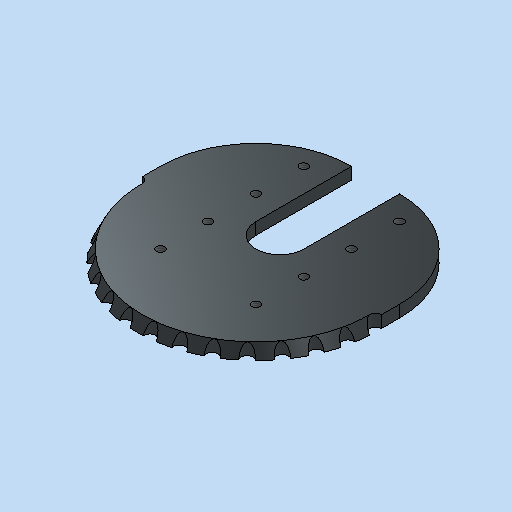
# Autodesk Inventor part: Blade
Saved by Autodesk Inventor 2026.1 (Build 301233000, 233)
## iProperties
Created: 2026-04-14
Part Number: Blade
Material: Iron, Gray
Document SubType Name: Modeling
Designer: ADMIN
Density: 7.15 g/cm^3
Appearance: Iron Gray
Author: ADMIN
Autodesk Inventor part; units mm, degrees
ref_plane "YZ Plane" through (0, 0, 0) normal (1, 0, 0) x (0, 1, 0)
ref_plane "XZ Plane" through (0, 0, 0) normal (0, 1, 0) x (-1, 0, 0)
ref_plane "XY Plane" through (0, 0, 0) normal (0, 0, 1) x (1, 0, 0)
sketch "Sketch1" plane through (0, 0, 0) normal (0, 1, 0) x (-1, 0, 0)
  line L0 (-10, -50) -> (10, -50)
  line L1 (50, -10) -> (50, 0)
  line L2 (0, 50) -> (0, 50)
  line L3 (-50, 0) -> (-50, -10)
  line L4 (-50, -50) -> (50, 50) construction
  line L5 (50, -50) -> (-50, 50) construction
  line L6 (-10, -50) -> (10, -50)
  line L7 (10, -50) -> (10, 0)
  line L8 (10, 0) -> (-10, 0)
  line L9 (-10, 0) -> (-10, -50)
  arc A0 (50, 0) -> (0, 50) centre (0, 0) ccw
  arc A1 (0, 50) -> (-50, 0) centre (0, 0) ccw
  arc A2 (10, -50) -> (50, -10) centre (10, -10) ccw
  arc A3 (-50, -10) -> (-10, -50) centre (-10, -10) ccw
  arc A4 (-50, -2.5) -> (-49.9375, 2.4992) centre (-50, 0) ccw
  line L10 (84.4975, 0) -> (-84.4975, 0) projected
  arc A5 (-49.4272, 7.9502) -> (-48.3266, 12.8272) centre (-48.9074, 10.3956) ccw
  arc A6 (-46.6941, 18.053) -> (-44.6037, 22.5946) centre (-45.6773, 20.3368) ccw
  arc A7 (-41.9203, 27.3667) -> (-38.9313, 31.3744) centre (-40.4508, 29.3893) ccw
  arc A8 (-35.3144, 35.4844) -> (-31.5574, 38.7831) centre (-33.4565, 37.1572) ccw
  arc A9 (-27.1651, 42.0513) -> (-22.8044, 44.4968) centre (-25, 43.3013) ccw
  arc A10 (-17.8285, 46.7803) -> (-13.0546, 48.2657) centre (-15.4508, 47.5528) ccw
  arc A11 (-7.7127, 49.4648) -> (-2.7344, 49.9252) centre (-5.2264, 49.7261) ccw
  arc A12 (2.7401, 49.9874) -> (7.7054, 49.4027) centre (5.2264, 49.7261) ccw
  arc A13 (13.0732, 48.3254) -> (17.8084, 46.7211) centre (15.4508, 47.5528) ccw
  arc A14 (22.8349, 44.5513) -> (27.1331, 41.9975) centre (25, 43.3013) ccw
  arc A15 (31.5987, 38.8301) -> (35.272, 35.4385) centre (33.4565, 37.1572) ccw
  arc A16 (38.9814, 31.4118) -> (41.8693, 27.3306) centre (40.4508, 29.3893) ccw
  arc A17 (44.6604, 22.6207) -> (46.6367, 18.0283) centre (45.6773, 20.3368) ccw
  arc A18 (48.3876, 12.841) -> (49.3659, 7.938) centre (48.9074, 10.3956) ccw
  arc A19 (50, 2.5) -> (49.9375, -2.4992) centre (50, 0) ccw
  circle A20 centre (20, -40) radius 1.75
  circle A21 centre (20, -20) radius 1.75
  circle A22 centre (20, 0) radius 1.75
  circle A23 centre (20, 20) radius 1.75
  line L11 (0, 50) -> (0, -50) construction
  circle A24 centre (-20, -40) radius 1.75
  circle A25 centre (-20, -20) radius 1.75
  circle A26 centre (-20, 0) radius 1.75
  circle A27 centre (-20, 20) radius 1.75
  line L12 (49.9375, -2.4992) -> (50, -2.4992)
  point P0 (0, 0)
  point P1 (47.5, 0)
  point P2 (49.9375, 2.4992)
  point P3 (49.3659, 7.938)
  point P4 (48.3266, 12.8272)
  point P5 (46.6367, 18.0283)
  point P6 (44.6037, 22.5946)
  point P7 (41.8693, 27.3306)
  point P8 (38.9313, 31.3744)
  point P9 (35.272, 35.4385)
  point P10 (31.5574, 38.7831)
  point P11 (27.1331, 41.9975)
  point P12 (22.8044, 44.4968)
  point P13 (17.8084, 46.7211)
  point P14 (13.0546, 48.2657)
  point P15 (2.7344, 49.9252)
  point P16 (0, 50)
  point P17 (-2.7344, 49.9252)
  point P18 (-7.7054, 49.4027)
  point P19 (-13.0546, 48.2657)
  point P20 (-17.8084, 46.7211)
  point P21 (-22.8044, 44.4968)
  point P22 (-27.1331, 41.9975)
  point P23 (-35.272, 35.4385)
  point P24 (-41.8693, 27.3306)
  point P25 (-44.6037, 22.5946)
  point P26 (-46.6367, 18.0283)
  point P27 (-48.3266, 12.8272)
  point P28 (-49.3659, 7.938)
  dimension "d0" = 100
  dimension "d1" = 100
  dimension "d2" = 20
  dimension "d3" = 50
  dimension "d4" = 50
  dimension "d5" = 40
  dimension "d6" = 5
  dimension "d9" = 180
  dimension "d11" = 3.5
  dimension "d12" = 3.5
  dimension "d13" = 3.5
  dimension "d14" = 3.5
  dimension "d15" = 20
  dimension "d16" = 20
  dimension "d17" = 20
  dimension "d18" = 10
  dimension "d19" = 10
  dimension "d20" = 10
  dimension "d21" = 10
  dimension "d22" = 10
  constraints: 42 point on circle, 28 centre point, 24 end point, 12 point on line, 8 tangent, 4 midpoint, 4 parallel, 4 symmetric about line, 3 perpendicular, 2 equal radius, 2 horizontal, 65 other
  measures "d0" distance of L5.start L4.end
  measures "d1" distance of L4.end L5.end
  measures "d2" distance of L7.end L8.end
  measures "d3" distance of L6.end L7.end
  measures "d4" radius of A0
  measures "d5" radius of A2
  measures "d6" diameter of A4
  measures "d11" diameter of A20
  measures "d12" diameter of A21
  measures "d13" diameter of A22
  measures "d14" diameter of A23
  measures "d15" distance of A20.centre A21.centre
  measures "d16" distance of A21.centre A22.centre
  measures "d17" distance of A23.centre A22.centre
  measures "d18" vertical distance of L11.end A20.centre
  measures "d19" distance from line of L7 A20.centre
  measures "d20" distance from line of L7 A21.centre
  measures "d21" distance from line of L7 A22.centre
  measures "d22" distance from line of L7 A23.centre
extrude "Extrusion1" add sketch "Sketch1" along normal blind 5 contours A3 L3 A4 L10 A26 L9 | L7 L10 A22 A19 L12 L1 A2 | L10 A26 A4 A1 A5 A6 A7 A8 A9 A10 A11 A0 A12 A13 A14 A15 A16 A17 A18 A19 A22 L8
sketch "Sketch2" plane through (0, 5, 0) normal (0, 1, 0) x (1, 0, 0)
  arc A0 (-10, 50) -> (-50, 10) centre (-10, 10) ccw projected
  line L0 (-50, 10) -> (-50, 2.4992) projected
  arc A1 (-49.9375, -2.4992) -> (-49.9375, 2.4992) centre (-50, 0) ccw projected
  arc A2 (-49.9375, -2.4992) -> (-49.3659, -7.938) centre (0, 0) ccw projected
  arc A3 (-48.3266, -12.8272) -> (-49.3659, -7.938) centre (-48.9074, -10.3956) ccw projected
  arc A4 (-48.3266, -12.8272) -> (-46.6367, -18.0283) centre (0, 0) ccw projected
  arc A5 (-44.6037, -22.5946) -> (-46.6367, -18.0283) centre (-45.6773, -20.3368) ccw projected
  arc A6 (-44.6037, -22.5946) -> (-41.8693, -27.3306) centre (0, 0) ccw projected
  arc A7 (-38.9313, -31.3744) -> (-41.8693, -27.3306) centre (-40.4508, -29.3893) ccw projected
  arc A8 (-38.9313, -31.3744) -> (-35.272, -35.4385) centre (0, 0) ccw projected
  arc A9 (-31.5574, -38.7831) -> (-35.272, -35.4385) centre (-33.4565, -37.1572) ccw projected
  arc A10 (-31.5574, -38.7831) -> (-27.1331, -41.9975) centre (0, 0) ccw projected
  arc A11 (-22.8044, -44.4968) -> (-27.1331, -41.9975) centre (-25, -43.3013) ccw projected
  arc A12 (-22.8044, -44.4968) -> (-17.8084, -46.7211) centre (0, 0) ccw projected
  arc A13 (-13.0546, -48.2657) -> (-17.8084, -46.7211) centre (-15.4508, -47.5528) ccw projected
  arc A14 (-13.0546, -48.2657) -> (-7.7054, -49.4027) centre (0, 0) ccw projected
  arc A15 (-2.7344, -49.9252) -> (-7.7054, -49.4027) centre (-5.2264, -49.7261) ccw projected
  arc A16 (-2.7344, -49.9252) -> (2.7344, -49.9252) centre (0, 0) ccw projected
  arc A17 (7.7054, -49.4027) -> (2.7344, -49.9252) centre (5.2264, -49.7261) ccw projected
  arc A18 (7.7054, -49.4027) -> (13.0546, -48.2657) centre (0, 0) ccw projected
  arc A19 (17.8084, -46.7211) -> (13.0546, -48.2657) centre (15.4508, -47.5528) ccw projected
  arc A20 (17.8084, -46.7211) -> (22.8044, -44.4968) centre (0, 0) ccw projected
  arc A21 (27.1331, -41.9975) -> (22.8044, -44.4968) centre (25, -43.3013) ccw projected
  arc A22 (27.1331, -41.9975) -> (31.5574, -38.7831) centre (0, 0) ccw projected
  arc A23 (35.272, -35.4385) -> (31.5574, -38.7831) centre (33.4565, -37.1572) ccw projected
  arc A24 (35.272, -35.4385) -> (38.9313, -31.3744) centre (0, 0) ccw projected
  arc A25 (41.8693, -27.3306) -> (38.9313, -31.3744) centre (40.4508, -29.3893) ccw projected
  arc A26 (41.8693, -27.3306) -> (44.6037, -22.5946) centre (0, 0) ccw projected
  arc A27 (46.6367, -18.0283) -> (44.6037, -22.5946) centre (45.6773, -20.3368) ccw projected
  arc A28 (46.6367, -18.0283) -> (48.3266, -12.8272) centre (0, 0) ccw projected
  arc A29 (49.3659, -7.938) -> (48.3266, -12.8272) centre (48.9074, -10.3956) ccw projected
  arc A30 (49.3659, -7.938) -> (49.9375, -2.4992) centre (0, 0) ccw projected
  arc A31 (50, 2.5) -> (49.9375, -2.4992) centre (50, 0) ccw projected
  line L1 (50, 2.5) -> (50, 10) projected
  arc A32 (50, 10) -> (10, 50) centre (10, 10) ccw projected
  line L2 (10, 50) -> (10, 0) projected
  line L3 (10, 0) -> (-10, 0) projected
  line L4 (-10, 0) -> (-10, 50) projected
  circle A33 centre (-20, 0) radius 1.75 projected
  circle A34 centre (-20, 40) radius 1.75 projected
  circle A35 centre (-20, 20) radius 1.75 projected
  circle A36 centre (20, 0) radius 1.75 projected
  circle A37 centre (20, 20) radius 1.75 projected
  circle A38 centre (20, 40) radius 1.75 projected
  circle A39 centre (-20, -20) radius 1.75 projected
  circle A40 centre (20, -20) radius 1.75 projected
  line L5 (-50, 2.4992) -> (-49.9375, 2.4992) projected
  line L6 (-47.5, 0) -> (47.5002, 0.0313)
  arc A41 (-47.5, 0) -> (47.5, 0.0313) centre (0, 0) ccw
  point P0 (0, 0)
  point P1 (-4.9651, -47.2398)
  constraints: 6 point on circle, 2 end point, 1 centre point, 1 coincident, 1 point on line
sketch "Sketch3" plane through (0, 0, 0) normal (0, 0, 1) x (1, 0, 0)
  line L0 (47.5, 5) -> (50, 0)
  line L1 (47.5, 0) -> (50, 0) projected
  line L2 (50, 0) -> (47.5, 0)
  line L3 (47.5, 0) -> (47.5, 5)
  line L4 (0, -1) -> (0, 6) projected
  line L5 (47.5, 5) -> (50, 5)
  line L6 (47.5, 5) -> (47.5, 0) projected
  line L7 (50, 0) -> (50, 5)
  point P0 (0, 0)
  point P1 (49.9375, 5)
  point P2 (49.9375, 0)
  constraints: 10 end point, 3 perpendicular, 1 collinear
revolve "Revolution1" cut sketch "Sketch3" angle 180 about axis through (0, -10, 0) along (0, -1, 0) contours L5 L7 L0
thread "Thread1" size "M5x0.8" class "6H" standard "ANSI Metric M Profile" full length
thread "Thread2" size "M5x0.8" class "6H" standard "ANSI Metric M Profile" full length
thread "Thread3" size "M5x0.8" class "6H" standard "ANSI Metric M Profile" full length
thread "Thread4" size "M5x0.8" class "6H" standard "ANSI Metric M Profile" full length
thread "Thread5" size "M5x0.8" class "6H" standard "ANSI Metric M Profile" full length
thread "Thread6" size "M5x0.8" class "6H" standard "ANSI Metric M Profile" full length
thread "Thread7" size "M5x0.8" class "6H" standard "ANSI Metric M Profile" full length
thread "Thread8" size "M5x0.8" class "6H" standard "ANSI Metric M Profile" full length
fillet "Fillet1" radius 10 2 edges at (-10, 2.5, 0) (10, 2.5, 0)
equation "\"d1\" = d0"
equation "\"d3\" = 0.5 * d0"
equation "\"d4\" = 0.5 * d0"
equation "\"d5\" = -0.5 * d2 + 0.5 * d0"
equation "\"d12\" = d11"
equation "\"d13\" = d11"
equation "\"d14\" = d11"
equation "\"d15\" = d2"
equation "\"d16\" = d15"
equation "\"d17\" = d15"
equation "\"d19\" = d18"
equation "\"d20\" = d19"
equation "\"d21\" = d19"
equation "\"d22\" = d19"
body "Solid1"
